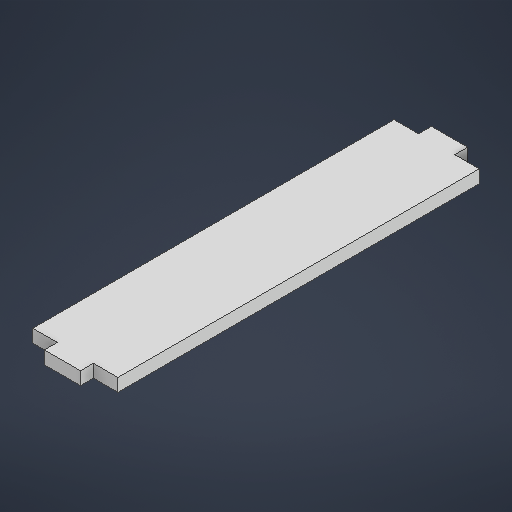
# Autodesk Inventor part: Part3
Saved by Autodesk Inventor 2027.1 (Build 311270010, 270A)
## iProperties
Created: 2026-10-07
Part Number: Part3
Material: Generic
Document SubType Name: Modeling
Designer: daniel
Density: 1 g/cm^3
Appearance: Default
Author: daniel
Autodesk Inventor part; units mm, degrees
ref_plane "YZ Plane" through (0, 0, 0) normal (1, 0, 0) x (0, 1, 0)
ref_plane "XZ Plane" through (0, 0, 0) normal (0, 1, 0) x (-1, 0, 0)
ref_plane "XY Plane" through (0, 0, 0) normal (0, 0, 1) x (1, 0, 0)
sketch "Sketch1" plane through (0, 0, 0) normal (0, 0, 1) x (1, 0, 0)
  line L0 (52.0118, 45.8669) -> (66.0118, 45.8669)
  line L1 (66.0118, 45.8669) -> (66.0118, 40.8669)
  line L2 (66.0118, 40.8669) -> (52.0118, 40.8669)
  line L3 (52.0118, 40.8669) -> (52.0118, 45.8669)
  line L4 (42.5118, 45.8669) -> (75.5118, 45.8669)
  line L5 (75.5118, 45.8669) -> (75.5118, 40.8669)
  line L6 (75.5118, 40.8669) -> (42.5118, 40.8669)
  line L7 (42.5118, 40.8669) -> (42.5118, 45.8669)
  point P0 (0, 0)
  point P1 (42.5118, 43.3669)
  point P2 (52.0118, 43.3669)
  dimension "d0" = 14
  dimension "d1" = 5
  dimension "d2" = 33
  dimension "d3" = 9.5
  constraints: 16 end point, 4 parallel, 2 horizontal, 2 midpoint, 2 perpendicular, 2 point on line
  measures "d0" distance of L1.end L2.end
  measures "d1" distance of L0.end L1.end
  measures "d2" distance of L5.end L6.end
  measures "d3" distance of point (42.512, 43.367) point (52.012, 43.367)
extrude "Extrusion1" add sketch "Sketch1" along normal mid plane 140
extrude "Extrusion2" add sketch "Sketch1" along normal mid plane 150 contours L0 L1 L2 L3
equation "\"d3\" = -0.5 * d0 + 0.5 * d2"
body "Solid1"
